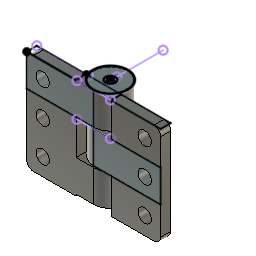
Parametric Hinge (Autodesk Fusion 360 design; units mm, degrees)
Autodesk Fusion 360 part; units mm, degrees
sketch "Central Hinge" plane through (0, 0, 0) normal (0, 0, 1) x (1, 0, 0)
  circle A0 centre (0, 0) radius 6.35
  circle A1 centre (0, 0) radius 1.5875
  circle A2 centre (0, 0) radius 1.8875
  circle A3 centre (0, 0) radius 6.65
  dimension "d10" = 12.7
  dimension "d11" = 3.175
  dimension "d12" = 3.775
  dimension "d35" = 13.3
  constraint coincident A0.centre A1.centre
  constraint concentric A0 A1
  constraint concentric A0 A3
  measures "d10" diameter of A0
  measures "d11" diameter of A1
  measures "d12" diameter of A2
  measures "d35" diameter of A3
extrude "Extrude1" add sketch "Central Hinge" against normal blind 12.1 from surface at -0.3 contours A0 makes body 1
ref_plane "WorkPlane1" through (0, -6.35, 0) normal (0, 1, 0) x (0, 0, 1)
pattern_linear "R-Pattern6" count 2 spacing 12.7 along (0, 0, -1) of bodies 1 makes body 2
sketch "Flats" plane through (0, -6.35, 0) normal (0, 1, 0) x (1, 0, 0)
  line L0 (0, 0.3) -> (-25.4, 0.3)
  line L1 (-25.4, 0.3) -> (-25.4, 12.4)
  line L2 (-25.4, 12.4) -> (0, 12.4)
  line L3 (0, 12.4) -> (0, 0.3)
  line L4 (-6.35, 0.3) -> (6.35, 0.3)
  line L5 (0, 13) -> (25.4, 13)
  line L6 (25.4, 13) -> (25.4, 25.1)
  line L7 (25.4, 25.1) -> (0, 25.1)
  line L8 (0, 25.1) -> (0, 13)
  line L9 (-6.35, 13) -> (6.35, 13)
  dimension "d30" = 25.4
  dimension "d31" = 12.1
  constraint horizontal L0
  constraint vertical L1
  constraint horizontal L2
  constraint vertical L3
  constraint midpoint L0.start L4
  constraint horizontal L5
  constraint vertical L6
  constraint horizontal L7
  constraint vertical L8
  constraint midpoint L5.start L9
  constraint equal L2 L7
  constraint equal L1 L6
  measures "d30" distance of L0.start L0.end
  measures "d31" distance of L0.end L1.end
extrude "Extrude2" add sketch "Flats" along normal blind 3.81 contours L0 L1 L2 L3 L4 bodies 1
pattern_linear "R-Pattern3" count 2 spacing 25.4 along (0, 0, -1) of bodies 1 makes body 3
sketch "Connectors" plane through (0, 0, -0.3) normal (0, 0, -1) x (1, 0, 0)
  line L0 (-25.4, 6.35) -> (-6.65, 6.35)
  line L1 (-6.65, 6.35) -> (-6.65, 2.54)
  line L2 (-6.65, 2.54) -> (-25.4, 2.54)
  line L3 (-25.4, 2.54) -> (-25.4, 6.35)
  line L4 (-25.4, 2.54) -> (-5.8199, 2.54)
  circle A0 centre (0, 0) radius 6.65
  line L5 (0, -2.5) -> (0, -20)
  line L6 (6.65, 2.54) -> (25.4, 2.54)
  line L7 (25.4, 6.35) -> (6.65, 6.35)
  line L8 (6.65, 6.35) -> (6.65, 2.54)
  line L9 (25.4, 2.54) -> (25.4, 6.35)
  line L10 (-6.65, 2.54) -> (6.65, 2.54)
  line L11 (6.65, 2.54) -> (6.65, 6.35)
  line L12 (6.65, 6.35) -> (-6.65, 6.35)
  line L13 (-6.65, 6.35) -> (-6.65, 2.54)
  point P0 (-25.4, 6.35)
  constraint horizontal L0
  constraint vertical L1
  constraint horizontal L2
  constraint vertical L3
  constraint coincident L1.end L4
  constraint coincident P0 L0.start
  constraint tangent L1 A0
  constraint symmetric P0 L5 L7.start
  constraint symmetric L0.end L5 L7.end
  constraint symmetric L1.end L5 L6.start
  constraint symmetric L2.end L5 L6.end
  constraint horizontal L10
  constraint vertical L11
  constraint horizontal L12
  constraint vertical L13
extrude "Extrude4" add sketch "Connectors" along normal blind 38.1 contours L0 L1 L2 L3 L4 L13 bodies 1 3
extrude "Extrude5" add sketch "Flats" along normal blind 3.81 contours L5 L6 L7 L8 L9 bodies 2
extrude "Extrude6" add sketch "Central Hinge" against normal up to surface (12.1 mm away) from surface at -13 contours A2 bodies 2
pattern_linear "R-Pattern4" count 1 spacing 25.4 along (0, 0, -1) of bodies 2 merged
extrude "Extrude7" add sketch "Connectors" along normal blind 38.1 contours L6 L7 L8 L9 L11 bodies 2
extrude "Extrude8" add sketch "Central Hinge" against normal blind 38.1 contours A1 bodies 2
sketch "Holes" plane through (0, -2.54, 0) normal (0, 1, 0) x (-1, 0, 0)
  line L0 (25.4, -0.3) -> (5.8199, -0.3)
  line L1 (5.8199, -0.3) -> (5.8199, -12.4)
  line L2 (5.8199, -12.4) -> (6.65, -12.4)
  line L3 (6.65, -12.4) -> (6.65, -25.7)
  line L4 (6.65, -38.4) -> (25.4, -38.4)
  line L5 (25.4, -38.4) -> (25.4, -0.3)
  circle A0 centre (19.35, -6.35) radius 2.54
  line L6 (25.4, -0.3) -> (25.4, -12.4)
  line L7 (25.4, -6.35) -> (19.35, -6.35)
  line L8 (0, 20) -> (0, 2.5)
  circle A1 centre (-19.35, -6.35) radius 2.54
  line L9 (6.65, -25.7) -> (5.8199, -25.7)
  line L10 (5.8199, -25.7) -> (5.8199, -37.8)
  line L11 (5.8199, -37.8) -> (6.65, -37.8)
  line L12 (6.65, -37.8) -> (6.65, -38.4)
  point P0 (6.65, -0.3)
  dimension "d57" = 5.08
  dimension "d59" = 12.7
  constraint midpoint L6 L7.start
  constraint coincident A0.centre L7.end
  constraint perpendicular L6 L7
  constraint symmetric A0 L8 A1
  measures "d57" diameter of A0
  measures "d59" horizontal distance of A0.centre P0
extrude "Extrude9" cut sketch "Holes" against normal up to surface (3.81 mm away) contours A0 | A1 bodies 1 2
pattern_linear "R-Pattern5" count 3 spacing 12.7 along (0, 0, -1) of "Extrude9"
fillet "Fillet1" radius 2.54 4 edges at (-25.4, -4.445, -0.3) (-25.4, -4.445, -38.4) (25.4, -4.445, -0.3) (25.4, -4.445, -38.4) on bodies 1 2
equation "WIDTH = 1 in" comment "Width of Hinge Plate"
equation "SPACING = 0.5 in" comment "Spacing of bolt holes"
equation "HOLE_DIAMETER = 0.2 in" comment "Diameter of bolt holes"
equation "HOLE_OFFSET = 0.5 in" comment "Offset from inside edge of hinge (noninterference at 270)"
equation "THICKNESS = 0.15 in" comment "Thickness of the hinge plates"
equation "AXIS_DIAMETER = 0.5 in" comment "Diameter of the hinge axis"
equation "ROD_DIAMETER = 0.125 in" comment "Diameter of the hinge rod"
equation "ROD_GAP = 0.3 mm" comment "Gap between Rod and Axis (will usually be doubled)"
equation "d10 = AXIS_DIAMETER"
equation "d11 = ROD_DIAMETER"
equation "d12 = ROD_DIAMETER + ROD_GAP * 2"
equation "d13 = -( SPACING - 2 * ROD_GAP )"
equation "NUM_HOLES = 3" comment "Number of holes (and hinge parts) minimum of 4"
equation "d20 = -ROD_GAP"
equation "SEGMENTS_A = floor(( NUM_HOLES + 1 ) / 2)" comment "Segments in part A"
equation "SEGMENTS_B = NUM_HOLES - SEGMENTS_A" comment "Segments in part B"
equation "d29 = -AXIS_DIAMETER / 2"
equation "d30 = WIDTH"
equation "d31 = SPACING - 2 * ROD_GAP"
equation "d32 = THICKNESS"
equation "d35 = AXIS_DIAMETER + ROD_GAP * 2"
equation "d36 = SEGMENTS_A"
equation "d38 = -SPACING * 2"
equation "d42 = NUM_HOLES * SPACING"
equation "d44 = THICKNESS"
equation "d49 = SEGMENTS_B"
equation "d51 = -SPACING * 2"
equation "d53 = NUM_HOLES * SPACING"
equation "d55 = -NUM_HOLES * SPACING"
equation "d57 = HOLE_DIAMETER"
equation "d59 = HOLE_OFFSET"
equation "d62 = NUM_HOLES"
equation "d64 = SPACING"
equation "d80 = -SPACING"
